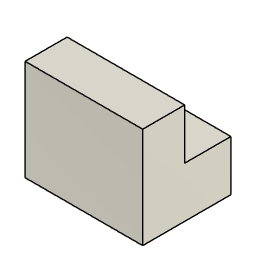
colour_detection_mechanism_top_panel_support (Autodesk Fusion 360 design; units mm, degrees)
part number: 2025-05-14-09-44-42-407
Autodesk Fusion 360 part; units mm, degrees
sketch "Sorting Mechanism Top Panel Support" plane through (0, 0, 0) normal (0, 0, 1) x (1, 0, 0)
  line L0 (0, 0) -> (28, 0)
  line L1 (28, 0) -> (28, 10)
  line L2 (28, 10) -> (0, 10)
  line L3 (0, 10) -> (0, 0)
  line L4 (28, 10) -> (0, 10)
  line L5 (0, 10) -> (0, 21)
  line L6 (0, 21) -> (28, 21)
  line L7 (28, 21) -> (28, 10)
  dimension "d1" = 10
  dimension "d2" = 28
  dimension "d5" = 11
  constraint horizontal L0
  constraint vertical L1
  constraint horizontal L2
  constraint vertical L3
  constraint coincident L0.start L3.end
  constraint horizontal L4
  constraint vertical L5
  constraint horizontal L6
  constraint vertical L7
  constraint collinear L3 L5
  measures "d1" distance of L0.end L1.end
  measures "d2" distance of L0.start L0.end
  measures "d5" distance of L1.end L6.end
extrude "Extrude1" add sketch "Sorting Mechanism Top Panel Support" along normal blind 24 contours L0 L1 L2 L3 L4
extrude "Extrude2" add sketch "Sorting Mechanism Top Panel Support" along normal blind 12 contours L2 L4 L5 L6 L7
named bodies: "Sorting Mechanism Top Panel Support"
